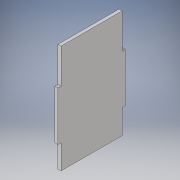
# Autodesk Inventor part: back
Saved by Autodesk Inventor 2017 (Build 210142000, 142)
## iProperties
Created: 2017-06-27
Part Number: back
Material: Generic
Document SubType Name: Modeling
Designer: millerid
Density: 1 g/cm^3
Appearance: Default
Author: millerid
Autodesk Inventor part; units mm, degrees
ref_plane "YZ Plane" through (0, 0, 0) normal (1, 0, 0) x (0, 1, 0)
ref_plane "XZ Plane" through (0, 0, 0) normal (0, 1, 0) x (-1, 0, 0)
ref_plane "XY Plane" through (0, 0, 0) normal (0, 0, 1) x (1, 0, 0)
sketch "Sketch1" plane through (0, 0, 0) normal (1, 0, 0) x (0, 1, 0)
  line L0 (0, 0) -> (25.2984, 0)
  line L1 (25.2984, 0) -> (25.2984, 3.175)
  line L2 (25.2984, 3.175) -> (76.3016, 3.175)
  line L3 (76.3016, 3.175) -> (76.3016, 0)
  line L4 (76.3016, 0) -> (112.395, 0)
  line L5 (112.395, 0) -> (112.395, -63.5)
  line L6 (112.395, -63.5) -> (76.3016, -63.5)
  line L7 (76.3016, -63.5) -> (76.3016, -66.675)
  line L8 (76.3016, -66.675) -> (25.2984, -66.675)
  line L9 (25.2984, -66.675) -> (25.2984, -63.5)
  line L10 (25.2984, -63.5) -> (0, -63.5)
  line L11 (0, -63.5) -> (0, 0)
  dimension "d0" = 25.2984
  dimension "d1" = 3.175
  dimension "d2" = 51.0032
  dimension "d3" = 63.5
  dimension "d4" = 3.175
  dimension "d5" = 112.395
  constraints: 24 end point, 7 perpendicular, 3 collinear, 2 horizontal, 2 point on line, 2 vertical
  measures "d0" distance of L0.start L0.end
  measures "d1" distance of L0.end L1.end
  measures "d2" distance of L1.end L2.end
  measures "d3" distance of L4.end L5.end
  measures "d4" distance of L6.end L7.end
  measures "d5" distance between parallel lines of L5 L11
extrude "Extrusion1" add sketch "Sketch1" along normal blind 3.175
body "Solid1"
